BasicRing v5 (Autodesk Fusion 360 design; units mm, degrees)
Autodesk Fusion 360 part; units mm, degrees
sketch "Sketch2" plane through (0, 0, 0) normal (0, 1, 0) x (1, 0, 0)
  circle A0 centre (0, 0) radius 32.5
  circle A1 centre (0, 0) radius 22.5
  dimension "d3" = 65
  dimension "d7" = -10
  constraint coincident A0.centre A1.centre
  measures "d3" diameter of A0
extrude "Extrude1" add sketch "Sketch2" along normal mid plane 4
sketch "Sketch1" plane through (0, 2, 0) normal (0, 1, 0) x (1, 0, 0)
  circle A0 centre (0, 27.5) radius 3.275
  circle A1 centre (0, 0) radius 22.5
  circle A2 centre (0, 0) radius 32.5
  line L0 (0, 32.5) -> (0, 27.5) construction
  line L1 (0, 27.5) -> (0, 22.5) construction
  dimension "d2" = 6.55
  constraint coincident A2 L0.start
  constraint coincident A0.centre L0.end
  constraint coincident A1 L1.end
  constraint equal L0 L1
  constraint collinear L0 L1
  constraint collinear A1.centre A0.centre L1.end
  constraint vertical L0
  measures "d2" diameter of A0
extrude "Extrude2" cut sketch "Sketch1" against normal through all contours A0
pattern_circular "C-Pattern1" count 3 over 360 about axis through (0, 2, 0) along (0, -1, 0) of "Extrude2"
equation "dowell_offset = 0.1 mm"
equation "d2 = dowell_diameter + ( 2 * dowell_offset )"
equation "d3 = ( 32.5 * 2 ) * 1 mm"
equation "dowell_diameter = ( 1 in / 4 in ) * 1 in"
